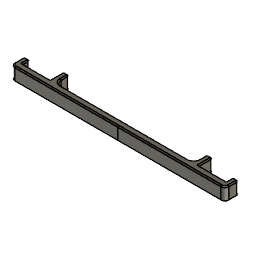
110mm_Y_alignment_spacer_x2 (Autodesk Fusion 360 design; units mm, degrees)
part number: 2026-06-27-10-18-24-577
Autodesk Fusion 360 part; units mm, degrees
other "Base Mesh Feature1"
sketch "Sketch1" plane through (0, 0, 0) normal (0, 0, 1) x (1, 0, 0)
  line L0 (-79.1, 5) -> (-75.1, 5)
  line L1 (-75.1, 0) -> (-75.1, 5)
  line L2 (-79.1, -5) -> (-79.1, 5)
  line L3 (-75.1, 0) -> (0, 0)
  line L4 (-79.1, -5) -> (0, -5)
  line L5 (-55, 10) -> (-55, 0)
  line L6 (-51, 10) -> (-51, 0)
  line L7 (-55, 10) -> (-51, 10)
  line L8 (0, -5) -> (0, 0)
  dimension "d1" = 5
  dimension "d2" = 4
  dimension "d3" = 10
  dimension "d4" = 20.1
  dimension "d5" = 4
  dimension "d6" = 10
  dimension "d18" = 55
  constraint horizontal L0
  constraint perpendicular L0 L1
  constraint perpendicular L0 L2
  constraint perpendicular L2 L3
  constraint horizontal L4
  constraint vertical L5
  constraint parallel L5 L6
  constraint horizontal L7
  constraint coincident L3 L6.end
  constraint coincident L3 L5.end
  constraint perpendicular L4 L8
  constraint coincident L3 L8.end
  constraint coincident L8 L3.end
  measures "d1" distance of L3 L4
  measures "d2" distance of L1 L2
  measures "d3" distance of L0 L4
  measures "d4" distance of L1 L5
  measures "d5" distance of L5 L6
  measures "d6" distance of L3 L7
  measures "d18" distance of L5 L8
extrude "Extrude1" add sketch "Sketch1" along normal blind 10
fillet "Fillet1" radius 3 1 edges at (-79.1, -5, 5)
fillet "Fillet1" radius 4 1 edges at (-51, 0, 5)
fillet "Fillet2" radius 1.2 2 edges at (-79.1, 5, 5) (-75.1, 5, 5)
fillet "Fillet2" radius 1.2 2 edges at (-55, 10, 5) (-51, 10, 5)
mirror "Mirror1" about plane through (0, 0, 0) normal (1, 0, 0) of bodies 1 merged
chamfer "Chamfer1" distance 0.8 angle 45 2 faces at (0, -1.6667, 10) (0, -1.6667, 0)
